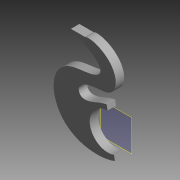
# Autodesk Inventor part: body06
Saved by Autodesk Inventor 2013 (Build 170138000, 138)
## iProperties
Created: 2013-02-19
Part Number: body06
Material: Generic
Document SubType Name: Modeling
Designer: Nano
Density: 1 g/cm^3
Author: Nano
Autodesk Inventor part; units mm, degrees
ref_plane "YZ Plane" through (0, 0, 0) normal (1, 0, 0) x (0, 1, 0)
ref_plane "XZ Plane" through (0, 0, 0) normal (0, 1, 0) x (-1, 0, 0)
ref_plane "XY Plane" through (0, 0, 0) normal (0, 0, 1) x (1, 0, 0)
ref_plane "Work Plane1" through (0, 0, -22.225) normal (0, 0, -1) x (-1, 0, 0)
sketch "Sketch1" plane through (0, 0, -22.225) normal (0, 0, -1) x (-1, 0, 0)
  arc A0 (-51.2256, -140.3966) -> (2.1978, 149.4337) centre (0, 0) ccw
  line L0 (-66.8621, -225.227) -> (19.0401, 240.8055) construction
  line L1 (-51.2256, -140.3966) -> (-58.4271, -179.4656)
  line L2 (2.1978, 149.4337) -> (9.7038, 190.1548)
  spline S0 degree 4 poles (-58.4271, -179.4656) (-17.1122, -200.4702) (126.981, -228.6588) (391.3947, -179.4269) (493.3076, 153.0777) (304.2628, 397.8504) (89.4201, 290.4612) (-75.3097, 427.2832) (304.6933, 583.1844) knots 0 0 0 0 0 0.221732 0.369889 0.516455 0.648201 1 1 1 1 1
  spline S1 degree 4 poles (9.7038, 190.1548) (69.4106, 178.9975) (139.3064, 136.1431) (235.6442, 109.8435) (261.3732, 230.4744) (95.7992, 280.8381) (-95.5214, 239.2892) (-108.3795, 542.1105) (151.6512, 607.836) (187.7745, 583.1844) knots 0 0 0 0 0 0.189742 0.310111 0.43027 0.567156 0.730861 1 1 1 1 1
  line L3 (187.7745, 583.1844) -> (304.6933, 583.1844)
  line L4 (-151.1409, -132.3296) -> (34.2867, -226.6016) construction
  arc A1 (-109.4654, -129.419) -> (12.0821, -191.2141) centre (-4.5292, -73.4516) ccw construction
  line L5 (-97.3852, 210.1664) -> (116.7928, 170.1432) construction
  arc A2 (88.9949, 162.2457) -> (-74.3153, 192.7632) centre (-40.724, -79.702) ccw construction
  line L6 (158.3267, 603.2804) -> (217.2224, 563.0885) construction
  arc A3 (196.6783, 566.7781) -> (169.2514, 585.4949) centre (176.2652, 566.3191) ccw construction
  point P0 (106.1828, -206.2676)
  point P1 (367.6104, -96.7927)
  point P2 (440.7438, 164.6389)
  point P3 (334.8261, 301.9441)
  point P4 (187.7745, 334.9467)
  point P5 (226.3731, 149.4344)
  point P6 (236.7093, 200.4766)
  point P7 (130.7306, 260.0966)
  point P8 (-26.7686, 294.7693)
  point P9 (-39.4608, 472.6968)
  point P10 (164.267, 138.3717)
  point P11 (75.1095, 372.2537)
  constraints: 14 end point, 6 midpoint, 5 point on circle, 4 centre point, 4 coincident, 4 point on line, 1 horizontal, 22 other
extrude "Extrusion1" add sketch "Sketch1" against normal blind 69.85
body "Solid1"
